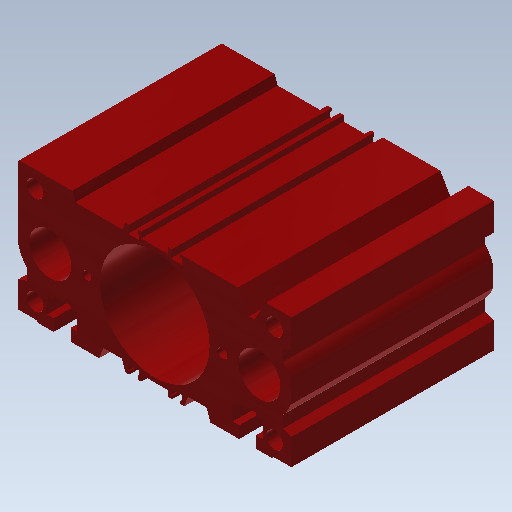
# Autodesk Inventor part: ADSK-MH-10029
Saved by Autodesk Inventor 2020.2 (Build 242310000, 310)
## iProperties
Created: 2008-03-10
Part Number: ADSK-MH-10029
Document SubType Name: Modeling
Designer: R.O'mahony
Density: 2.71 g/cm^3
Mass: 2122.1 g
Surface Area: 1595.47 cm^2
Volume: 783.065 cm^3
Material: Aluminum 6061
Appearance: Red
Description: Pneumatic Housing
Engineer: Demir Ali
Checked By: Demir Ali
Company: Autodesk Ltd
Author: R.O'mahony
Keywords: Roller Conveyor
Revision Number: A
Autodesk Inventor part; units mm, degrees
ref_plane "YZ Plane" through (0, 0, 0) normal (1, 0, 0) x (0, 1, 0)
ref_plane "XZ Plane" through (0, 0, 0) normal (0, 1, 0) x (-1, 0, 0)
ref_plane "XY Plane" through (0, 0, 0) normal (0, 0, 1) x (1, 0, 0)
sketch "Sketch1" plane through (0, 0, 0) normal (0, 0, 1) x (1, 0, 0)
  line L0 (2486.1475, -489.1271) -> (2514.8357, -489.1271)
  line L1 (2487.5916, -556.1271) -> (2483.6916, -556.1271)
  line L2 (2483.6916, -546.1271) -> (2487.5916, -546.1271)
  line L3 (2486.5114, -490.1271) -> (2484.6916, -485.1271)
  line L4 (2483.6916, -563.1271) -> (2500.6916, -563.1271)
  line L5 (2454.6916, -545.8991) -> (2454.6916, -533.6796)
  line L6 (2457.6916, -537.7009) -> (2457.6916, -544.8072)
  line L7 (2483.6916, -559.1271) -> (2473.6916, -559.1271)
  arc A0 (2469.7916, -554.0046) -> (2472.6916, -546.1271) centre (2468.6916, -549.1271) ccw
  line L8 (2473.6916, -544.6271) -> (2483.6916, -544.6271)
  line L9 (2469.7916, -546.1271) -> (2473.6916, -546.1271)
  line L10 (2469.7916, -556.1271) -> (2469.7916, -546.1271)
  line L11 (2473.6916, -556.1271) -> (2469.7916, -556.1271)
  line L12 (2473.6916, -563.1271) -> (2473.6916, -556.1271)
  line L13 (2483.6916, -556.1271) -> (2483.6916, -563.1271)
  line L14 (2483.6916, -544.6271) -> (2483.6916, -546.1271)
  line L15 (2457.6916, -544.8072) -> (2452.6916, -546.6271)
  line L16 (2473.6916, -546.1271) -> (2473.6916, -544.6271)
  line L17 (2463.8276, -562.1271) -> (2464.1916, -563.1271)
  line L18 (2452.6916, -562.1271) -> (2463.8276, -562.1271)
  line L19 (2452.6916, -546.6271) -> (2452.6916, -562.1271)
  line L20 (2464.1916, -563.1271) -> (2473.6916, -563.1271)
  circle A1 centre (2462.6916, -553.1271) radius 5
  circle A2 centre (2471.6916, -524.1271) radius 12.5
  circle A3 centre (2471.6916, -524.1271) radius 12
  arc A4 (2452.6916, -528.5146) -> (2457.6916, -537.7009) centre (2471.6916, -524.1271) ccw
  arc A5 (2453.6916, -485.1271) -> (2452.6916, -486.1271) centre (2453.6916, -486.1271) ccw
  line L21 (2452.6916, -486.1271) -> (2452.6916, -528.5146)
  line L22 (2484.6916, -485.1271) -> (2453.6916, -485.1271)
  circle A6 centre (2462.6916, -495.1271) radius 5
  line L23 (2612.6916, -533.6796) -> (2612.6916, -545.8991)
  line L24 (2609.6916, -544.8072) -> (2609.6916, -537.7009)
  circle A7 centre (2533.6916, -524.1271) radius 32.5
  line L25 (2593.6916, -559.1271) -> (2583.6916, -559.1271)
  line L26 (2583.6916, -544.6271) -> (2593.6916, -544.6271)
  line L27 (2541.6916, -559.1271) -> (2525.6916, -559.1271)
  line L28 (2515.0177, -559.1271) -> (2502.1475, -559.1271)
  line L29 (2524.1616, -559.1271) -> (2517.8616, -559.1271)
  line L30 (2518.5116, -562.6271) -> (2516.2916, -562.6271)
  line L31 (2523.5116, -560.8271) -> (2523.5116, -562.6271)
  line L32 (2518.5116, -562.6271) -> (2518.5116, -560.8271)
  line L33 (2525.6916, -559.1271) -> (2525.6916, -562.6271)
  line L34 (2525.6916, -562.6271) -> (2523.5116, -562.6271)
  line L35 (2487.5916, -546.1271) -> (2487.5916, -556.1271)
  line L36 (2524.1616, -560.8271) -> (2523.5116, -560.8271)
  line L37 (2524.1616, -557.6271) -> (2524.1616, -560.8271)
  line L38 (2517.8616, -557.6271) -> (2524.1616, -557.6271)
  line L39 (2517.8616, -560.8271) -> (2517.8616, -557.6271)
  line L40 (2518.5116, -560.8271) -> (2517.8616, -560.8271)
  line L41 (2514.1078, -556.6271) -> (2516.2916, -562.6271)
  line L42 (2503.0574, -556.6271) -> (2514.1078, -556.6271)
  line L43 (2500.6916, -563.1271) -> (2503.0574, -556.6271)
  line L44 (2549.5216, -559.1271) -> (2543.2216, -559.1271)
  line L45 (2565.2357, -559.1271) -> (2552.3655, -559.1271)
  line L46 (2541.6916, -562.6271) -> (2541.6916, -559.1271)
  line L47 (2551.0916, -562.6271) -> (2548.8716, -562.6271)
  line L48 (2548.8716, -560.8271) -> (2548.8716, -562.6271)
  line L49 (2549.5216, -560.8271) -> (2548.8716, -560.8271)
  line L50 (2549.5216, -557.6271) -> (2549.5216, -560.8271)
  line L51 (2543.2216, -557.6271) -> (2549.5216, -557.6271)
  line L52 (2543.2216, -560.8271) -> (2543.2216, -557.6271)
  line L53 (2543.8716, -562.6271) -> (2541.6916, -562.6271)
  line L54 (2579.7916, -556.1271) -> (2579.7916, -546.1271)
  line L55 (2583.6916, -556.1271) -> (2579.7916, -556.1271)
  line L56 (2543.8716, -562.6271) -> (2543.8716, -560.8271)
  line L57 (2543.8716, -560.8271) -> (2543.2216, -560.8271)
  line L58 (2553.2754, -556.6271) -> (2564.3258, -556.6271)
  line L59 (2579.7916, -546.1271) -> (2583.6916, -546.1271)
  line L60 (2583.6916, -563.1271) -> (2583.6916, -556.1271)
  line L61 (2583.6916, -546.1271) -> (2583.6916, -544.6271)
  line L62 (2551.0916, -562.6271) -> (2553.2754, -556.6271)
  line L63 (2564.3258, -556.6271) -> (2566.6916, -563.1271)
  line L64 (2566.6916, -563.1271) -> (2583.6916, -563.1271)
  arc A8 (2593.6916, -549.1271) -> (2597.5916, -554.0046) centre (2598.6916, -549.1271) ccw
  arc A9 (2594.6916, -546.1271) -> (2593.6916, -549.1271) centre (2598.6916, -549.1271) ccw
  line L65 (2593.6916, -556.1271) -> (2593.6916, -563.1271)
  line L66 (2597.5916, -556.1271) -> (2593.6916, -556.1271)
  line L67 (2597.5916, -546.1271) -> (2597.5916, -556.1271)
  line L68 (2593.6916, -546.1271) -> (2597.5916, -546.1271)
  line L69 (2603.5556, -562.1271) -> (2614.6916, -562.1271)
  line L70 (2614.6916, -546.6271) -> (2609.6916, -544.8072)
  line L71 (2603.1916, -563.1271) -> (2603.5556, -562.1271)
  line L72 (2593.6916, -544.6271) -> (2593.6916, -546.1271)
  line L73 (2593.6916, -563.1271) -> (2603.1916, -563.1271)
  line L74 (2614.6916, -562.1271) -> (2614.6916, -546.6271)
  circle A10 centre (2604.6916, -553.1271) radius 5
  line L75 (2585.001, -489.1271) -> (2597.3822, -489.1271)
  circle A11 centre (2595.6916, -524.1271) radius 12.5
  circle A12 centre (2595.6916, -524.1271) radius 12
  line L76 (2592.7634, -497.1271) -> (2589.6198, -497.1271)
  line L77 (2541.6916, -489.1271) -> (2525.6916, -489.1271)
  line L78 (2517.8616, -489.1271) -> (2524.1616, -489.1271)
  line L79 (2525.6916, -485.6271) -> (2523.5116, -485.6271)
  line L80 (2524.1616, -490.6271) -> (2524.1616, -487.4271)
  line L81 (2524.1616, -487.4271) -> (2523.5116, -487.4271)
  line L82 (2523.5116, -487.4271) -> (2523.5116, -485.6271)
  line L83 (2518.5116, -485.6271) -> (2516.1096, -485.6271)
  line L84 (2525.6916, -489.1271) -> (2525.6916, -485.6271)
  line L85 (2518.5116, -485.6271) -> (2518.5116, -487.4271)
  line L86 (2518.5116, -487.4271) -> (2517.8616, -487.4271)
  line L87 (2517.8616, -487.4271) -> (2517.8616, -490.6271)
  line L88 (2517.8616, -490.6271) -> (2524.1616, -490.6271)
  line L89 (2516.1096, -485.6271) -> (2514.4717, -490.1271)
  line L90 (2514.4717, -490.1271) -> (2486.5114, -490.1271)
  circle A13 centre (2493.6916, -524.1271) radius 2.5
  line L91 (2543.2216, -489.1271) -> (2549.5216, -489.1271)
  arc A14 (2573.6916, -521.6271) -> (2573.6916, -526.6271) centre (2573.6916, -524.1271) ccw
  arc A15 (2573.6916, -526.6271) -> (2573.6916, -521.6271) centre (2573.6916, -524.1271) ccw
  line L92 (2589.6198, -497.1271) -> (2582.9803, -485.6271)
  line L93 (2543.8716, -487.4271) -> (2543.2216, -487.4271)
  line L94 (2543.2216, -487.4271) -> (2543.2216, -490.6271)
  line L95 (2543.2216, -490.6271) -> (2549.5216, -490.6271)
  line L96 (2582.9803, -485.6271) -> (2548.8716, -485.6271)
  line L97 (2541.6916, -485.6271) -> (2541.6916, -489.1271)
  line L98 (2549.5216, -487.4271) -> (2548.8716, -487.4271)
  line L99 (2548.8716, -487.4271) -> (2548.8716, -485.6271)
  line L100 (2543.8716, -485.6271) -> (2543.8716, -487.4271)
  line L101 (2549.5216, -490.6271) -> (2549.5216, -487.4271)
  line L102 (2543.8716, -485.6271) -> (2541.6916, -485.6271)
  line L103 (2573.1916, -526.6271) -> (2574.1916, -526.6271)
  arc A16 (2573.1916, -521.6271) -> (2573.1916, -526.6271) centre (2573.1916, -524.1271) ccw
  line L104 (2574.1916, -521.6271) -> (2573.1916, -521.6271)
  arc A17 (2574.1916, -526.6271) -> (2574.1916, -521.6271) centre (2574.1916, -524.1271) ccw
  line L105 (2612.6916, -502.355) -> (2612.6916, -514.5746)
  line L106 (2599.6916, -485.1271) -> (2592.7634, -497.1271)
  line L107 (2609.6916, -503.4469) -> (2614.6916, -501.6271)
  line L108 (2609.6916, -510.5532) -> (2609.6916, -503.4469)
  arc A18 (2609.6916, -537.7009) -> (2614.1916, -530.2915) centre (2595.6916, -524.1271) ccw
  arc A19 (2614.1916, -517.9627) -> (2609.6916, -510.5532) centre (2595.6916, -524.1271) ccw
  line L109 (2614.1916, -530.2915) -> (2614.1916, -517.9627)
  line L110 (2613.6916, -485.1271) -> (2599.6916, -485.1271)
  arc A20 (2614.6916, -486.1271) -> (2613.6916, -485.1271) centre (2613.6916, -486.1271) ccw
  circle A21 centre (2604.6916, -495.1271) radius 5
  line L111 (2614.6916, -501.6271) -> (2614.6916, -486.1271)
  point P0 (0, 0)
  dimension "d2" = 124
  constraints: 224 end point, 27 point on circle, 27 point on line, 22 centre point, 2 midpoint
  measures "d2" distance of A11.centre A2.centre
extrude "Extrusion1" add sketch "Sketch1" along normal blind 120 contours L3 L90 L89 L83 L85 L86 L87 L88 L80 L81 L82 L79 L84 L77 L97 L102 L100 L93 L94 L95 L101 L98 L99 L96 L92 L76 L106 L110 A20 L111 L107 L108 A19 L109 A18 L24 L70 L74 L69 L71 L73 L65 L66 L67 L68 L72 L26 L61 L59 L54 L55 L60 L64 L63 L58 L62 L47 L48 L49 L50 L51 L52 L57 L56 L53 L46 L27 L33 L34 L31 L36 L37 L38 L39 L40 L32 L30 L41 L42 L43 L4 L13 L1 L35 L2 L14 L8 L16 L9 L10 L11 L12 L20 L17 L18 L19 L15 L6 A4 L21 A5 L22
body "Solid1"
